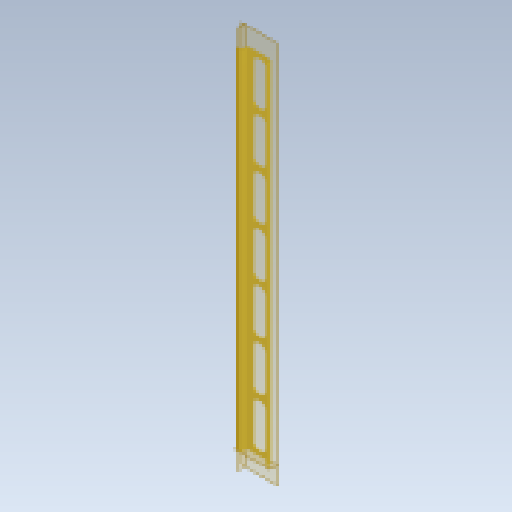
# Autodesk Inventor part: PP0735H(1)
Saved by Autodesk Inventor 2025.2 (Build 292293000, 293)
## iProperties
Category: PARTsolutions
Company: ELDON
Created: 2025-05-02
Part Number: PP0735H(1)
Material: Ouro
Catalog Web Link: www.cadenas.de
Description: PP-DIN rails
Vendor: ELDON
Document SubType Name: Modeling
Designer: psAdmin
Manufacturer: ELDON
Mass: 630 g
Surface Area: 1764.71 cm^2
Volume: 84.5125 cm^3
Density: 19.3 g/cm^3
Appearance: Metal quente 2400F
PSOL_IDENT_0: {$CADENAS_DATA/23d-libs/eldon/common_pool/accessories/p/pp.prj},167 {VTYP=3D},{NB=PP0735H(1)},{LINA=
PSOL_IDENT_1: PP0735H},{NN=PP},{DATE=04.03.2025 09:38:01},{GEOMDATE=28.02.2025 11:58:07},{VERSION=},{LINEID=1810},
PSOL_IDENT_2: {WBVAR=DETAIL},{WBNUMERIC=DETAIL}  {NB=PP0735H(1)},{LINA=PP0735H},{KT=DUMMY},{ITEM=PP0735H},{DETAIL=
PSOL_IDENT_3: 1},{INFO=Info URL},{DES=Din rail with holes, 2000},{DES1=With holes},{MAT=Galvanized steel},{TYP=Ome
PSOL_IDENT_4: ga},{DIM=7.5 X 35},{HP=Hole pattern 18 x 5.2 mm},{MASS=0.63},{EAN=8713574013193},{TARIFFN=-},{MI=URL
PSOL_IDENT_5: },{MIALG=https://www.eldon.com/catalog-document/PP0515H/mountinginstructions/en/},{INFOPATH=https://
PSOL_IDENT_6: www.nvent.com/en-gb/catalog-document/itemsheet?pid=PP0735H},{V=1},{A=35},{A1=7.5},{A2=4.00},{A3=0.8}
PSOL_IDENT_7: ,{A4=1.8},{A5=0.00},{A6=0.0}
NB: PP0735H(1)
NN: PP
NT: DIN rails
NBSYN: $ITEM.($DETAIL.)
LINA: PP0735H
CATALOG: nVent HOFFMAN IEC-Rated Products
ITEM: PP0735H
DETAIL: high
INFO: Info URL
DES: Din rail with holes, 2000
DES1: With holes
MAT: Galvanized steel
TYP: Omega
DIM: 7.5 X 35
HP: Hole pattern 18 x 5.2 mm
MASS: 0.63
EAN: 8713574013193
MI: URL
SUPPLIER: ELDON
ARTICLENO: PP0735H(1)
BOMINFO: PP0735H
CREATOR: CADENAS GmbH
Title: PP0735H
Author: Cadenas PARTsolutions
Comments: DIN rails
Autodesk Inventor part; units mm, degrees
sketch "Sketch_2" plane through (0, 0, 0) normal (0, 1, 0) x (-1, 0, 0)
  line L0 (0.7786, 2.7778) -> (0.7786, 3.2051)
  line L1 (0.7786, 3.2051) -> (-0.5889, 3.2051)
  arc A0 (-0.5889, 3.2051) -> (-1.3581, 2.4359) centre (-0.5889, 2.4359) ccw
  line L2 (-1.3581, 2.4359) -> (-1.3581, 0.7692)
  arc A1 (-1.7, 0.4274) -> (-1.3581, 0.7692) centre (-1.7, 0.7692) ccw
  line L3 (-1.7, 0.4274) -> (-11.7, 0.4274)
  arc A2 (-12.0419, 0.7692) -> (-11.7, 0.4274) centre (-11.7, 0.7692) ccw
  line L4 (-12.0419, 0.7692) -> (-12.0419, 2.4359)
  arc A3 (-12.0419, 2.4359) -> (-12.8111, 3.2051) centre (-12.8111, 2.4359) ccw
  line L5 (-12.8111, 3.2051) -> (-14.1786, 3.2051)
  line L6 (-14.1786, 3.2051) -> (-14.1786, 2.7778)
  line L7 (-14.1786, 2.7778) -> (-12.8111, 2.7778)
  arc A4 (-12.4692, 2.4359) -> (-12.8111, 2.7778) centre (-12.8111, 2.4359) ccw
  line L8 (-12.4692, 2.4359) -> (-12.4692, 0.7692)
  arc A5 (-12.4692, 0.7692) -> (-11.7, 0) centre (-11.7, 0.7692) ccw
  line L9 (-11.7, 0) -> (-1.7, 0)
  arc A6 (-1.7, 0) -> (-0.9308, 0.7692) centre (-1.7, 0.7692) ccw
  line L10 (-0.9308, 0.7692) -> (-0.9308, 2.4359)
  arc A7 (-0.5889, 2.7778) -> (-0.9308, 2.4359) centre (-0.5889, 2.4359) ccw
  line L11 (-0.5889, 2.7778) -> (0.7786, 2.7778)
  dimension "d14" = 10
  constraints: 24 end point, 16 point on circle, 8 centre point, 5 equal radius, 1 parallel
  measures "d14" distance of L9.start L9.end
extrude "Extrusion1" add sketch "Sketch_2" along normal blind 159
sketch "Sketch_6" plane through (0, 0, 0) normal (0, 0, 1) x (1, 0, 0)
  arc A0 (4.05, 4.6232) -> (9.95, 4.6232) centre (7, 4.6232) ccw
  line L0 (9.95, 4.6232) -> (9.95, 19.1463)
  arc A1 (9.95, 19.1463) -> (4.05, 19.1463) centre (7, 19.1463) ccw
  line L1 (4.05, 19.1463) -> (4.05, 4.6232)
  dimension "d13" = 2.95
  constraints: 4 end point, 4 point on circle, 2 centre point, 1 equal radius
  measures "d13" radius of A0
extrude "Extrusion2" cut sketch "Sketch_6" along normal blind 2
pattern_linear "Rectangular Pattern1" count 80 spacing 22.6 along (0, 1, 0) of "Extrusion2"
body "Solid1"
